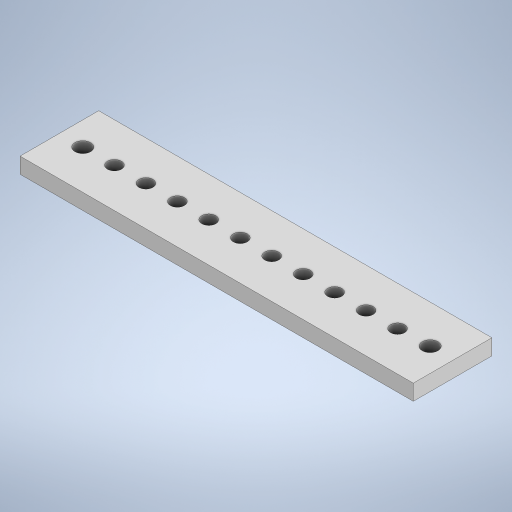
# Autodesk Inventor part: Busbar Copper
Saved by Autodesk Inventor 2023 (Build 270158000, 158)
## iProperties
Created: 2023-03-08
Part Number: Busbar Copper
Material: Generic
Document SubType Name: Modeling
Designer: cheng
Density: 1 g/cm^3
Appearance: Default
Author: cheng
Autodesk Inventor part; units mm, degrees
ref_plane "YZ Plane" through (0, 0, 0) normal (1, 0, 0) x (0, 1, 0)
ref_plane "XZ Plane" through (0, 0, 0) normal (0, 1, 0) x (-1, 0, 0)
ref_plane "XY Plane" through (0, 0, 0) normal (0, 0, 1) x (1, 0, 0)
sketch "Sketch1" plane through (0, 0, 0) normal (0, 1, 0) x (-1, 0, 0)
  line L0 (25, -5) -> (-25, -5)
  line L1 (-25, -5) -> (-25, 5)
  line L2 (-25, 5) -> (25, 5)
  line L3 (25, 5) -> (25, -5)
  line L4 (25, -5) -> (-25, 5) construction
  line L5 (-25, -5) -> (25, 5) construction
  point P0 (0, 0)
  dimension "d0" = 10
  dimension "d1" = 50
  constraints: 12 end point, 2 midpoint, 2 parallel, 1 horizontal, 1 perpendicular
  measures "d0" distance between parallel lines of L2 L0
  measures "d1" distance between parallel lines of L1 L3
extrude "Extrusion1" add sketch "Sketch1" along normal blind 2
sketch "Sketch2" plane through (0, 2, 0) normal (0, 1, 0) x (1, 0, 0)
  line L0 (-25, -5) -> (25, -5) projected
  line L1 (25, -5) -> (25, 5) projected
  line L2 (25, 5) -> (-25, 5) projected
  line L3 (-25, 5) -> (-25, -5) projected
  line L4 (-25, 0) -> (25, 0)
  line L5 (0, 5) -> (0, -5)
  point P0 (0, 0)
  point P1 (-18, 0)
  point P2 (18, 0)
  dimension "d11" = 18
  dimension "d12" = 18
  constraints: 4 end point, 4 midpoint, 1 point on line
  measures "d11" distance from line of L5 point (-18, 0)
  measures "d12" distance from line of L5 point (18, 0)
hole "Hole1" at (-18, 2, 0) at (18, 2, 0) direction (0, -1, 0) diameter 1.778 end through all
sketch "Sketch3" plane through (0, 2, 0) normal (0, 1, 0) x (1, 0, 0)
  circle A0 centre (-18, 0) radius 0.889 projected
  circle A1 centre (18, 0) radius 0.889 projected
  line L0 (-25, -5) -> (25, -5) projected
  line L1 (25, -5) -> (25, 5) projected
  line L2 (25, 5) -> (-25, 5) projected
  line L3 (-25, 5) -> (-25, -5) projected
  line L4 (-25, 0) -> (25, 0) construction
  line L5 (0, 5) -> (0, -5) construction
  point P0 (0, 0)
  point P1 (14, 0)
  point P2 (-14, 0)
  point P3 (-10, 0)
  point P4 (-6, 0)
  point P5 (-2, 0)
  point P6 (2, 0)
  point P7 (6, 0)
  point P8 (10, 0)
  dimension "d21" = 4
  dimension "d22" = 4
  dimension "d23" = 4
  dimension "d24" = 2
  dimension "d25" = 2
  dimension "d26" = 4
  dimension "d27" = 4
  dimension "d28" = 4
  constraints: 4 midpoint, 2 end point, 11 other
  measures "d21" distance of point (-10, 0) point (-14, 0)
  measures "d22" distance of point (-6, 0) point (-10, 0)
  measures "d23" distance of point (-2, 0) point (-6, 0)
  measures "d24" distance from line of L5 point (-2, 0)
  measures "d25" distance from line of L5 point (2, 0)
  measures "d26" distance of point (2, 0) point (6, 0)
  measures "d27" distance of point (6, 0) point (10, 0)
  measures "d28" distance of point (10, 0) point (14, 0)
hole "Hole2" at (14, 2, 0) at (-14, 2, 0) at (-10, 2, 0) at (-6, 2, 0) at (-2, 2, 0) at (2, 2, 0) at (6, 2, 0) at (10, 2, 0) direction (0, -1, 0) diameter 1.778 end through all
sketch "Sketch4" plane through (0, 2, 0) normal (0, 1, 0) x (1, 0, 0)
  circle A0 centre (6, 0) radius 0.889 projected
  circle A1 centre (-2, 0) radius 0.889 projected
  circle A2 centre (-10, 0) radius 0.889 projected
  circle A3 centre (14, 0) radius 0.889 projected
  circle A4 centre (-14, 0) radius 0.889 projected
  circle A5 centre (-6, 0) radius 0.889 projected
  circle A6 centre (2, 0) radius 0.889 projected
  circle A7 centre (10, 0) radius 0.889 projected
  circle A8 centre (-18, 0) radius 0.889 projected
  circle A9 centre (18, 0) radius 0.889 projected
  line L0 (-25, -5) -> (25, -5) projected
  line L1 (25, -5) -> (25, 5) projected
  line L2 (25, 5) -> (-25, 5) projected
  line L3 (-25, 5) -> (-25, -5) projected
  line L4 (-25, 0) -> (25, 0) construction
  point P0 (0, 0)
  point P1 (-22, -0.0247)
  point P2 (22, 0.138)
  dimension "d37" = 4
  dimension "d38" = 4
  constraints: 2 end point, 2 midpoint
  measures "d37" horizontal distance of A8.centre point (-22, -0.025)
  measures "d38" horizontal distance of A9.centre point (22, 0.138)
hole "Hole3" at (-22, 2, 0.0247) at (22, 2, -0.138) direction (0, -1, 0) diameter 2 end through all
equation "\"d38\" = d37"
body "Solid1"
